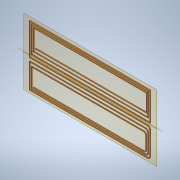
# Autodesk Inventor part: primary_coil_0R2
Saved by Autodesk Inventor 2021 (Build 250183000, 183)
## iProperties
Created: 2021-01-20
Part Number: primary_coil_0R2
Material: Generic
Document SubType Name: Modeling
Designer: phamv
Density: 1 g/cm^3
Appearance: Default
Author: phamv
Autodesk Inventor part; units mm, degrees
ref_plane "YZ Plane" through (0, 0, 0) normal (1, 0, 0) x (0, 1, 0)
sketch "Sketch1" plane through (0, 0, 0) normal (0, 0, 1) x (1, 0, 0)
  line L0 (0, -9.3) -> (385, -9.3)
  line L1 (400, -24.3) -> (400, -185)
  line L2 (385, -200) -> (-400, -200)
  line L3 (-400, -200) -> (-400, -32.4)
  line L4 (0, -9.3) -> (0, -13.8)
  line L5 (0, -13.8) -> (380.5, -13.8)
  line L6 (395.5, -28.8) -> (395.5, -180.5)
  line L7 (380.5, -195.5) -> (-395.5, -195.5)
  line L8 (-400, -32.4) -> (372.25, -32.4)
  line L9 (387.25, -47.4) -> (387.25, -172.25)
  line L10 (372.25, -187.25) -> (-387.25, -187.25)
  line L11 (-395.5, -195.5) -> (-395.5, -36.9)
  line L12 (-395.5, -36.9) -> (367.75, -36.9)
  line L13 (382.75, -51.9) -> (382.75, -167.75)
  line L14 (367.75, -182.75) -> (-382.75, -182.75)
  line L15 (-382.75, -182.75) -> (-382.75, -60)
  line L16 (-387.25, -187.25) -> (-387.25, -55.5)
  line L17 (-387.25, -55.5) -> (359.5, -55.5)
  line L18 (374.5, -70.5) -> (374.5, -159.5)
  line L19 (-382.75, -60) -> (355, -60)
  line L20 (370, -75) -> (370, -155)
  line L21 (-560.8284, 0) -> (564.9706, 0) projected
  line L22 (355, -170) -> (-374.5, -170)
  line L23 (359.5, -174.5) -> (-374.5, -174.5)
  line L24 (-374.5, -174.5) -> (-374.5, -170)
  arc A0 (400, -24.3) -> (385, -9.3) centre (385, -24.3) ccw
  arc A1 (395.5, -28.8) -> (380.5, -13.8) centre (380.5, -28.8) ccw
  arc A2 (387.25, -47.4) -> (372.25, -32.4) centre (372.25, -47.4) ccw
  arc A3 (382.75, -51.9) -> (367.75, -36.9) centre (367.75, -51.9) ccw
  arc A4 (374.5, -70.5) -> (359.5, -55.5) centre (359.5, -70.5) ccw
  arc A5 (370, -75) -> (355, -60) centre (355, -75) ccw
  arc A6 (355, -170) -> (370, -155) centre (355, -155) ccw
  arc A7 (359.5, -174.5) -> (374.5, -159.5) centre (359.5, -159.5) ccw
  arc A8 (367.75, -182.75) -> (382.75, -167.75) centre (367.75, -167.75) ccw
  arc A9 (372.25, -187.25) -> (387.25, -172.25) centre (372.25, -172.25) ccw
  arc A10 (380.5, -195.5) -> (395.5, -180.5) centre (380.5, -180.5) ccw
  arc A11 (385, -200) -> (400, -185) centre (385, -185) ccw
  point P0 (0, 0)
  point P1 (400, -9.3)
  point P2 (400, -200)
  point P3 (395.5, -13.8)
  point P4 (395.5, -195.5)
  point P5 (387.25, -32.4)
  point P6 (387.25, -187.25)
  point P7 (382.75, -36.9)
  point P8 (382.75, -182.75)
  point P9 (374.5, -55.5)
  point P10 (374.5, -174.5)
  point P11 (370, -60)
  point P12 (370, -170)
  point P13 (0, 0)
  dimension "d1" = 4.5
  dimension "d2" = 4.5
  dimension "d3" = 4.5
  dimension "d4" = 9.3
  dimension "d5" = 800
  dimension "d6" = 400
  dimension "d7" = 4.5
  dimension "d8" = 4.5
  dimension "d9" = 8.25
  dimension "d10" = 4.5
  dimension "d11" = 18.6
  dimension "d12" = 4.5
  dimension "d13" = 8.25
  dimension "d14" = 4.5
  dimension "d15" = 4.5
  dimension "d16" = 4.5
  dimension "d17" = 8.25
  dimension "d19" = 18.6
  dimension "d20" = 8.25
  dimension "d82" = 200
  dimension "d88" = 4.5
  dimension "d89" = 8.25
  dimension "d90" = 8.25
  dimension "d91" = 15
  constraints: 48 end point, 24 point on circle, 24 point on line, 24 tangent, 15 perpendicular, 12 centre point, 11 equal radius, 4 horizontal, 3 vertical, 2 parallel, 1 coincident
  measures "d1" distance between parallel lines of L5 L0
  measures "d2" distance between parallel lines of L6 L1
  measures "d3" distance between parallel lines of L2 L7
  measures "d4" distance from line of L21 L0.start
  measures "d5" distance between parallel lines of L3 L1
  measures "d6" distance from line of point (0, 0) L1
  measures "d7" distance between parallel lines of L3 L11
  measures "d8" distance between parallel lines of L13 L9
  measures "d9" distance between parallel lines of L9 L6
  measures "d10" distance between parallel lines of L8 L12
  measures "d11" distance between parallel lines of L8 L5
  measures "d12" distance between parallel lines of L10 L14
  measures "d13" distance between parallel lines of L7 L10
  measures "d14" distance between parallel lines of L16 L15
  measures "d15" distance between parallel lines of L17 L19
  measures "d16" distance between parallel lines of L20 L18
  measures "d17" distance between parallel lines of L18 L13
  measures "d19" distance between parallel lines of L17 L12
  measures "d20" distance between parallel lines of L11 L16
  measures "d82" distance between parallel lines of L2 L21
  measures "d88" distance between parallel lines of L23 L22
  measures "d89" distance between parallel lines of L14 L23
  measures "d90" distance between parallel lines of L15 L24
  measures "d91" radius of A0
extrude "Extrusion1" add sketch "Sketch1" along normal blind 4.5
sketch "Sketch3" plane through (0, 0, 0) normal (0, 0, 1) x (1, 0, 0)
  line L0 (0, -13.8) -> (-400, -13.8)
  line L1 (-400, -13.8) -> (-400, 200)
  line L2 (-400, 200) -> (400, 200)
  line L3 (400, 200) -> (400, 9.3)
  line L4 (0, -9.3) -> (-395.5, -9.3)
  line L5 (-395.5, -9.3) -> (-395.5, 195.5)
  line L6 (-395.5, 195.5) -> (395.5, 195.5)
  line L7 (395.5, 195.5) -> (395.5, 13.8)
  line L8 (395.5, 13.8) -> (-382.75, 13.8)
  line L9 (-382.75, 13.8) -> (-382.75, 182.75)
  line L10 (400, 9.3) -> (-387.25, 9.3)
  line L11 (-387.25, 9.3) -> (-387.25, 187.25)
  line L12 (-382.75, 182.75) -> (382.75, 182.75)
  line L13 (-387.25, 187.25) -> (387.25, 187.25)
  line L14 (382.75, 182.75) -> (382.75, 36.9)
  line L15 (382.75, 36.9) -> (-370, 36.9)
  line L16 (387.25, 187.25) -> (387.25, 32.4)
  line L17 (387.25, 32.4) -> (-374.5, 32.4)
  line L18 (-370, 36.9) -> (-370, 170)
  line L19 (-370, 170) -> (373.75, 170)
  line L20 (373.75, 170) -> (373.75, 60)
  line L21 (373.75, 60) -> (-361.75, 60)
  line L22 (-374.5, 32.4) -> (-374.5, 174.5)
  line L23 (-374.5, 174.5) -> (378.25, 174.5)
  line L24 (378.25, 174.5) -> (378.25, 55.5)
  line L25 (378.25, 55.5) -> (-361.75, 55.5)
  line L26 (-361.75, 60) -> (-361.75, 55.5)
  line L27 (400, -185) -> (400, -24.3) projected
  line L28 (-560, 0) -> (560, 0) projected
  point P0 (0, 0)
  point P1 (0, 200)
  point P2 (400, -200)
  point P3 (400, -9.3)
  dimension "d58" = 4.5
  dimension "d59" = 4.5
  dimension "d60" = 4.5
  dimension "d61" = 8.25
  dimension "d62" = 8.25
  dimension "d64" = 4.5
  dimension "d65" = 4.5
  dimension "d66" = 4.5
  dimension "d67" = 8.25
  dimension "d68" = 800
  dimension "d69" = 18.6
  dimension "d70" = 4.5
  dimension "d71" = 4.5
  dimension "d72" = 18.6
  dimension "d73" = 8.25
  dimension "d74" = 8.25
  dimension "d75" = 4.5
  dimension "d76" = 4.5
  dimension "d77" = 18.6
  dimension "d78" = 4.5
  dimension "d79" = 4.5
  dimension "d80" = 4.5
  dimension "d83" = 200
  dimension "d87" = 8.25
  constraints: 54 end point, 16 perpendicular, 4 parallel, 3 horizontal, 3 vertical, 1 collinear, 1 midpoint, 1 other
  measures "d58" distance between parallel lines of L1 L5
  measures "d59" distance between parallel lines of L2 L6
  measures "d60" distance between parallel lines of L7 L3
  measures "d61" distance between parallel lines of L13 L6
  measures "d62" distance between parallel lines of L5 L11
  measures "d64" distance between parallel lines of L10 L8
  measures "d65" distance between parallel lines of L14 L16
  measures "d66" distance between parallel lines of L13 L12
  measures "d67" distance between parallel lines of L16 L7
  measures "d68" distance between parallel lines of L1 L3
  measures "d69" distance between parallel lines of L4 L10
  measures "d70" distance between parallel lines of L11 L9
  measures "d71" distance between parallel lines of L17 L15
  measures "d72" distance between parallel lines of L8 L17
  measures "d73" distance between parallel lines of L12 L23
  measures "d74" distance between parallel lines of L9 L22
  measures "d75" distance between parallel lines of L23 L19
  measures "d76" distance between parallel lines of L24 L14
  measures "d77" distance between parallel lines of L15 L25
  measures "d78" distance between parallel lines of L24 L20
  measures "d79" distance between parallel lines of L25 L21
  measures "d80" distance between parallel lines of L22 L18
  measures "d83" distance of the line from the sketch origin of L2
  measures "d87" distance between parallel lines of L18 L26
extrude "Extrusion2" add sketch "Sketch3" along normal blind 4.5 fills toward (-197.75, -9.35) open curves L4 L5 L6 L7 L8 L9 L12 L14 L15 L18 L19 L20 L21 L26 L25 L24 L23 L22 L17 L16 L13 L11 L10 L3 L2 L1 L0
equation "\"d1\" = wire_diameter"
equation "\"d2\" = wire_diameter"
equation "\"d3\" = wire_diameter"
equation "\"d4\" = 0.5 * distance_between_wires"
equation "\"d5\" = track_length"
equation "\"d6\" = 0.5 * track_length"
equation "\"d7\" = wire_diameter"
equation "\"d8\" = wire_diameter"
equation "\"d9\" = distance_between_wires_edge"
equation "\"d10\" = wire_diameter"
equation "\"d11\" = distance_between_wires"
equation "\"d12\" = wire_diameter"
equation "\"d13\" = distance_between_wires_edge"
equation "\"d14\" = wire_diameter"
equation "\"d15\" = wire_diameter"
equation "\"d16\" = wire_diameter"
equation "\"d17\" = distance_between_wires_edge"
equation "\"d19\" = distance_between_wires"
equation "\"d20\" = distance_between_wires_edge"
equation "\"d82\" = 0.5 * track_width"
equation "\"d22\" = wire_diameter"
equation "\"d58\" = wire_diameter"
equation "\"d59\" = wire_diameter"
equation "\"d60\" = wire_diameter"
equation "\"d61\" = distance_between_wires_edge"
equation "\"d62\" = distance_between_wires_edge"
equation "\"d64\" = wire_diameter"
equation "\"d65\" = wire_diameter"
equation "\"d66\" = wire_diameter"
equation "\"d67\" = distance_between_wires_edge"
equation "\"d68\" = track_length"
equation "\"d69\" = distance_between_wires"
equation "\"d70\" = wire_diameter"
equation "\"d71\" = wire_diameter"
equation "\"d72\" = distance_between_wires"
equation "\"d73\" = distance_between_wires_edge"
equation "\"d74\" = distance_between_wires_edge"
equation "\"d75\" = wire_diameter"
equation "\"d76\" = wire_diameter"
equation "\"d77\" = distance_between_wires"
equation "\"d78\" = wire_diameter"
equation "\"d79\" = wire_diameter"
equation "\"d80\" = wire_diameter"
equation "\"d83\" = 0.5 * track_width"
equation "\"d85\" = wire_diameter"
equation "\"track_length\" = 800"
equation "\"wire_diameter\" = 4.5"
equation "\"distance_between_wires\" = -1.2 * wire_diameter + 0.2 * parameter_6"
equation "\"distance_between_wires_edge\" = 8.25"
equation "\"d84\" = wire_diameter"
equation "\"bend_radius\" = 15"
equation "\"track_width\" = 400"
equation "\"parameter_6\" = 120"
body "Solid1"
